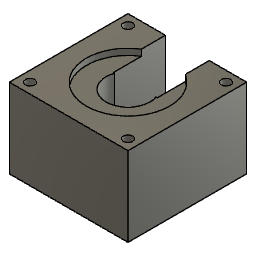
BearingBlock v18 (Autodesk Fusion 360 archive; units mm, degrees)
design "BearingBlock" references "tormach 770mx"
Autodesk Fusion 360 part; units mm, degrees
sketch "Sketch1" plane through (0, 0, 0) normal (0, 1, 0) x (1, 0, 0)
  line L0 (0, 0) -> (57.1, 0)
  line L1 (57.1, 0) -> (57.1, -57.1)
  line L2 (57.1, -57.1) -> (0, -57.1)
  line L3 (0, -57.1) -> (0, 0)
  dimension "d1" = 57.1
  dimension "d28" = 57.1
  constraint horizontal L0
  constraint vertical L1
  constraint horizontal L2
  constraint vertical L3
  constraint coincident L0.start L3.end
  measures "d1" distance of L0.start L0.end
  measures "d28" distance of L0 L2
extrude "Extrude1" add sketch "Sketch1" along normal blind 38.2
sketch "Sketch2" plane through (0, 38.2, 0) normal (0, 1, 0) x (-1, 0, 0)
  line L0 (0, 57.1) -> (-57.1, 57.1)
  line L1 (-57.1, 57.1) -> (-57.1, 0)
  line L2 (-57.1, 0) -> (0, 0)
  line L3 (0, 0) -> (0, 57.1)
  line L4 (0, 28.55) -> (-57.1, 28.55) construction
  line L5 (-28.55, 0) -> (-28.55, 57.1) construction
  circle A0 centre (-28.55, 28.55) radius 20
  line L6 (-4.98, 52.12) -> (-52.12, 52.12) construction
  line L7 (-52.12, 52.12) -> (-52.12, 4.98) construction
  line L8 (-52.12, 4.98) -> (-4.98, 4.98) construction
  line L9 (-4.98, 4.98) -> (-4.98, 52.12) construction
  line L10 (-4.98, 52.12) -> (-52.12, 4.98) construction
  line L11 (-52.12, 52.12) -> (-4.98, 4.98) construction
  point P0 (-28.55, 28.55)
  point P1 (-28.55, 28.55)
  point P2 (-52.12, 4.98)
  point P3 (-4.98, 4.98)
  point P4 (-4.98, 52.12)
  point P5 (-52.12, 52.12)
  dimension "d7" = 40
  dimension "d14" = 47.14
  dimension "d15" = 47.14
  constraint midpoint L3 L4.start
  constraint midpoint L1 L4.end
  constraint midpoint L2 L5.start
  constraint midpoint L0 L5.end
  constraint midpoint L4 P1
  constraint coincident P1 P0
  constraint horizontal L6
  constraint perpendicular L6 L7
  constraint parallel L6 L8
  constraint parallel L7 L9
  constraint coincident L10 P1
  constraint coincident L11 P1
  constraint coincident P2 L7.end
  constraint coincident P3 L8.end
  constraint coincident P4 L6.start
  constraint coincident P5 L6.end
  measures "d7" diameter of A0
  measures "d14" distance of P2 P3
  measures "d15" distance of P5 P2
hole "Hole1" at (28.55, 38.2, 28.55) direction (0, -1, 0) diameter 21.1 end through all
extrude "Extrude2" cut sketch "Sketch2" against normal blind 3 contours A0
sketch "Sketch3" plane through (0, 0, 0) normal (0, -1, 0) x (1, 0, 0)
  circle A0 centre (28.55, 28.55) radius 10.55
  line L0 (57.1, 57.1) -> (0, 57.1)
  line L1 (0, 57.1) -> (0, 0)
  line L2 (0, 0) -> (57.1, 0)
  line L3 (57.1, 0) -> (57.1, 57.1)
  circle A1 centre (28.55, 28.55) radius 11.125
  line L4 (18.0066, 25) -> (39.0934, 25)
  line L5 (39.0934, 25) -> (39.0934, 0)
  line L6 (39.0934, 0) -> (18.0066, 0)
  line L7 (18.0066, 0) -> (18.0066, 25)
  arc A2 (39.0934, 25) -> (28.55, 17.425) centre (28.55, 28.55) ccw
  arc A3 (18.6152, 25) -> (38.4848, 25) centre (28.55, 28.9746) ccw
  dimension "d11" = 22.25
  dimension "d41" = 25
  constraint concentric A0 A1
  constraint horizontal L4
  constraint vertical L5
  constraint horizontal L6
  constraint vertical L7
  constraint coincident L2 L5.end
  constraint coincident A1 L4.start
  constraint coincident A1 L4.end
  constraint coincident L4.start A2
  constraint coincident A1 A2.end
  constraint tangent A2 A3
  constraint coincident L4 A3.end
  constraint coincident A0 A3.end
  constraint coincident L4 A3.start
  constraint coincident A0 A3.start
  measures "d11" diameter of A1
  measures "d41" distance of L4.start L6.end
extrude "Extrude3" cut sketch "Sketch3" against normal blind 0.65 contours A0 A1 L4 A2 | A0 A1 L4 A2
hole "Hole6" at (4.98, 38.2, 4.98) direction (0, -1, 0) diameter 4.5 end through all
hole "Hole7" at (52.12, 38.2, 4.98) direction (0, -1, 0) diameter 4.5 end through all
hole "Hole8" at (52.12, 38.2, 52.12) direction (0, -1, 0) diameter 4.5 end through all
hole "Hole9" at (4.98, 38.2, 52.12) direction (0, -1, 0) diameter 4.5 end through all
extrude "Extrude4" cut sketch "Sketch3" against normal through all contours L2 A1 L5 L6 L7 A2
extrude "Extrude5" cut sketch "Sketch3" against normal blind 38 contours A0 A1 L4 A2 | L4 A3 picked at (28.55, 17.8267)
fillet "Fillet1" [rolled back] radius 3
